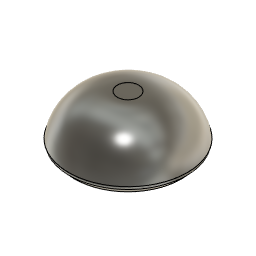
Topper - large dome v3 (Autodesk Fusion 360 design; units mm, degrees)
Autodesk Fusion 360 part; units mm, degrees
sketch "Sketch1" plane through (0, 0, 0) normal (0, 1, 0) x (1, 0, 0)
  line L0 (0, 0) -> (7, 0)
  line L1 (7, 0) -> (7, -4)
  line L2 (7, -4) -> (17, -4)
  line L3 (0, -18) -> (0, 0)
  line L4 (0, -18) -> (3, -18)
  arc A0 (3, -18) -> (17, -4) centre (3, -4) ccw
  dimension "d1" = 7
  dimension "d2" = 4
  dimension "d3" = 10
  dimension "d4" = 3
  dimension "d5" = 18
  constraint coincident L0.start L3.end
  constraint horizontal L0
  constraint perpendicular L0 L1
  constraint perpendicular L1 L2
  constraint perpendicular L0 L3
  constraint perpendicular L3 L4
  constraint tangent L4 A0
  measures "d1" distance of L0.start L0.end
  measures "d2" distance of L0.end L1.end
  measures "d3" distance of L1.end L2.end
  measures "d4" distance of L3.start L4.end
  measures "d5" distance of L3.start L0.start
revolve "Revolve1" add sketch "Sketch1" angle 360 about axis through (0, 0, 18) along (0, 0, -1)
sketch "Sketch2" plane through (0, 0, 0) normal (0, 0, -1) x (1, 0, 0)
  circle A0 centre (0, 0) radius 7
  line L0 (1.55, 1.05) -> (1.55, -1.05)
  line L1 (-1.55, 1.05) -> (-1.55, -1.05)
  line L2 (0.55, -2.05) -> (-0.55, -2.05)
  line L3 (0.55, 2.05) -> (-0.55, 2.05)
  arc A1 (0.55, -2.05) -> (1.55, -1.05) centre (0.55, -1.05) ccw
  arc A2 (-0.55, 2.05) -> (-1.55, 1.05) centre (-0.55, 1.05) ccw
  arc A3 (-1.55, -1.05) -> (-0.55, -2.05) centre (-0.55, -1.05) ccw
  arc A4 (1.55, 1.05) -> (0.55, 2.05) centre (0.55, 1.05) ccw
  point P0 (0, -2.05)
  point P1 (1.55, 2.05)
  point P2 (1.55, -2.05)
  point P3 (1.55, 0)
  point P4 (-1.55, 2.05)
  dimension "d11" = 4.1
  dimension "d12" = 3.1
  dimension "d13" = 1
  constraint vertical L1
  constraint vertical L0
  constraint horizontal A0.centre P3
  constraint coincident A0.centre origin
  constraint horizontal L2
  constraint horizontal L3
  constraint vertical A0.centre P0
  constraint coincident P0 L2
  constraint coincident P3 L0
  constraint coincident P2 L2
  constraint coincident P2 L0
  constraint tangent L2 A1
  constraint tangent L0 A1
  constraint coincident P4 L3
  constraint coincident P4 L1
  constraint tangent L3 A2
  constraint tangent L1 A2
  constraint equal A1 A2
  constraint tangent L2 A3
  constraint tangent L1 A3
  constraint equal A1 A3
  constraint coincident P1 L0
  constraint coincident P1 L3
  constraint tangent L0 A4
  constraint tangent L3 A4
  constraint equal A1 A4
  constraint midpoint P0 L2
  constraint midpoint P3 L0
  measures "d11" distance of P1 P2
  measures "d12" distance of P1 P4
  measures "d13" radius of A1
extrude "Extrude1" cut sketch "Sketch2" against normal blind 2.5 contours L0 L1 L2 L3 A1 A2 A3 A4
chamfer "Chamfer1" distance 2 angle 45 1 edges at (-15.8496, -6.1475, 4)
fillet "Fillet1" radius 1 1 edges at (15.7164, -6.0958, 5.9949)
